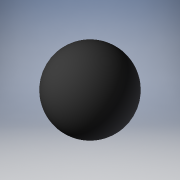
# Autodesk Inventor part: 51110 Ball
Saved by Autodesk Inventor 2019 (Build 230136000, 136)
## iProperties
Created: 2023-07-26
Part Number: 51110 Ball
Material: Generic
Catalog Web Link: www.cadenas.de
Description: With flat seet B-
Vendor: NSK_RB
Document SubType Name: Modeling
Designer: psAdmin
Manufacturer: NSK_RB
Mass: 0.179594 g
Surface Area: 1.53938 cm^2
Volume: 0.179594 cm^3
Density: 1 g/cm^3
Appearance: PSOLRGB-175-175-175
Category: PARTsolutions
Company: NSK_RB
Title: 51110 Ball
Author: Cadenas PARTsolutions
PSOL_IDENT_0: {$CADENAS_DATA/23d-libs/nsk_rb/roller_bearings/thrust_bearings/single_direction_tbb/with_flat_seet_b
PSOL_IDENT_1: .prj},172 {VTYP=3D},{NB=51110 Ball},{LINA=51110 Ball},{NN=With flat seet B},{DATE=27.09.2022 23:23:1
PSOL_IDENT_2: 0},{GEOMDATE=02.08.2010 09:29:00},{VERSION=},{LINEID=6550},{WBVAR=},{WBNUMERIC=}  {NB=51110 Ball},{L
PSOL_IDENT_3: INA=51110 Ball},{KT=DUMMY},{IDNR=},{STAN=},{NO=31},{ORDER=51110},{SD=50},{D=70},{T=14},{T3=0.0},{T4=
PSOL_IDENT_4: 0},{SR=0.6},{CAN=29000},{COAN=75500},{CA=2960},{COA=7700},{GRE=3200},{OIL=4800},{SD1=70},{D1=52},{D2=
PSOL_IDENT_5: 0},{D3=0},{SB=0.0},{A=0.0},{R=0},{SDA=62},{DA=58},{SRA=0.6},{MASS=0.153},{N=10}
NB: 51110 Ball
NN: With flat seet B
NBSYN: $ORDER. Ball
LINA: 51110 Ball
CATALOG: NSK Rolling Bearing
NO: 31
ORDER: 51110
SD: 50
D: 70
T: 14
T3: 0
T4: 0
SR: 0.6
CAN: 29000
COAN: 75500
CA: 2960
COA: 7700
GRE: 3200
OIL: 4800
SD1: 70
D1: 52
D2: 0
D3: 0
SB: 0
A: 0
R: 0
SDA: 62
DA: 58
SRA: 0.6
MASS: 0.153
N: 10
SUPPLIER: NSK_RB
ARTICLENO: 51110 Ball
BOMINFO: 51110 Ball
CREATOR: CADENAS GmbH
Autodesk Inventor part; units mm, degrees
sketch "Sketch_1" plane through (0, 0, 0) normal (0, 0, 1) x (1, 0, 0)
  line L0 (3.5, 0) -> (-3.5, 0)
  arc A0 (3.5, 0) -> (-3.5, 0) centre (0, 0) ccw
  line L1 (3.5, 0) -> (-3.5, 0)
  constraints: 4 end point, 2 point on circle, 1 centre point
revolve "Revolution1" add sketch "Sketch_1" angle 360 about axis through (3.5, 0, 0) along (1, 0, 0)
ref_plane "B_HW_XY" through (0, 0, 0) normal (1, 0, 0) x (0, 0, -1)
ref_plane "B_HW_YZ" through (0, 0, 0) normal (0, 0, -1) x (0, 1, 0)
ref_plane "B_HW_ZX" through (0, 0, 0) normal (0, 1, 0) x (1, 0, 0)
body "Solid1"
